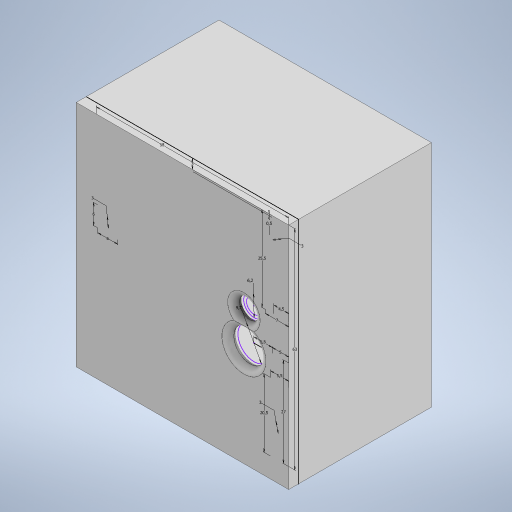
# Autodesk Inventor part: slave2
Saved by Autodesk Inventor 2023 (Build 270158000, 158)
## iProperties
Created: 2023-12-13
Part Number: slave2
Material: Generic
Document SubType Name: Modeling
Designer: magnu
Density: 1 g/cm^3
Appearance: Default
Author: magnu
Autodesk Inventor part; units mm, degrees
ref_plane "YZ Plane" through (0, 0, 0) normal (1, 0, 0) x (0, 1, 0)
ref_plane "XZ Plane" through (0, 0, 0) normal (0, 1, 0) x (-1, 0, 0)
ref_plane "XY Plane" through (0, 0, 0) normal (0, 0, 1) x (1, 0, 0)
sketch "Sketch1" plane through (0, 0, 0) normal (0, 0, 1) x (1, 0, 0)
  line L0 (0, 0) -> (58, 0)
  line L1 (58, 0) -> (58, 63)
  line L2 (58, 63) -> (0, 63)
  line L3 (0, 63) -> (0, 0)
  line L4 (0.5, 62.5) -> (57.5, 62.5)
  line L5 (57.5, 62.5) -> (57.5, 0.5)
  line L6 (57.5, 0.5) -> (0.5, 0.5)
  line L7 (0.5, 0.5) -> (0.5, 62.5)
  circle A0 centre (54.5, 8.5) radius 1.5
  circle A1 centre (54.5, 57.5) radius 1.5
  circle A2 centre (3.5, 36.5) radius 1.5
  line L8 (-3, 66) -> (61, 66)
  line L9 (61, 66) -> (61, -3)
  line L10 (61, -3) -> (-3, -3)
  line L11 (-3, -3) -> (-3, 66)
  line L12 (58, 63) -> (51, 63)
  line L13 (51, 63) -> (51, 37.5)
  line L14 (51, 37.5) -> (58, 37.5)
  line L15 (58, 37.5) -> (58, 63)
  line L16 (58, 0) -> (52.5, 0)
  line L17 (52.5, 0) -> (52.5, 20.5)
  line L18 (52.5, 20.5) -> (58, 20.5)
  line L19 (58, 20.5) -> (58, 0)
  line L20 (58, 20.5) -> (53.5, 20.5)
  line L21 (53.5, 20.5) -> (53.5, 37.5)
  line L22 (53.5, 37.5) -> (58, 37.5)
  line L23 (58, 37.5) -> (58, 20.5)
  line L24 (58, 0) -> (58, 27)
  line L25 (58, 27) -> (53, 27)
  line L26 (53, 27) -> (47.5, 27)
  circle A3 centre (47.5, 36.75) radius 2.25
  line L27 (51, 37.5) -> (51, 32.1962)
  line L28 (51, 21.8038) -> (52.5, 20.5)
  circle A4 centre (47.5, 27) radius 4.85
  circle A5 centre (47.5, 36.75) radius 3.1
  circle A6 centre (47.5, 27) radius 6
  line L29 (51, 34.1296) -> (51, 31.8734)
  line L30 (51, 21.8038) -> (50.7926, 21.9841)
  line L31 (6.5, 39.5) -> (0.5, 39.5)
  line L32 (0.5, 39.5) -> (0.5, 33.5)
  line L33 (0.5, 33.5) -> (6.5, 33.5)
  line L34 (6.5, 33.5) -> (6.5, 39.5)
  line L35 (6.5, 39.5) -> (0.5, 33.5) construction
  line L36 (0.5, 39.5) -> (6.5, 33.5) construction
  line L37 (6.5, 39.5) -> (0, 39.5)
  line L38 (0, 39.5) -> (0, 33.5)
  line L39 (0, 33.5) -> (6.5, 33.5)
  line L40 (6.5, 33.5) -> (6.5, 39.5)
  point P0 (52.5, 0.5)
  point P1 (51, 62.5)
  point P2 (50.5, 37.531)
  point P3 (50.5, 35.969)
  point P4 (57.5, 20.5)
  point P5 (57.5, 37.5)
  dimension "d0" = 58
  dimension "d1" = 63
  dimension "d2" = 0.5
  dimension "d3" = 3
  dimension "d4" = 3
  dimension "d5" = 3
  dimension "d6" = 3
  dimension "d11" = 7
  dimension "d12" = 25.5
  dimension "d13" = 5.5
  dimension "d14" = 20.5
  dimension "d15" = 4.5
  dimension "d16" = 27
  dimension "d17" = 5
  dimension "d18" = 5.5
  dimension "d25" = 9.7
  dimension "d26" = 6.2
  dimension "d31" = 6
  dimension "d32" = 6
  constraints: 82 end point, 16 parallel, 9 perpendicular, 8 point on line, 7 centre point, 6 horizontal, 2 coincident, 2 midpoint, 2 point on circle, 1 vertical, 6 other
  measures "d0" distance of L2.end L1.end
  measures "d1" distance of L1.end L0.end
  measures "d2" distance between parallel lines of L2 L4
  measures "d3" diameter of A0
  measures "d4" diameter of A1
  measures "d5" diameter of A2
  measures "d6" distance between parallel lines of L2 L8
  measures "d11" distance of L14.end L13.end
  measures "d12" distance of L13.end L12.end
  measures "d13" distance of L17.end L18.end
  measures "d14" distance of L16.end L17.end
  measures "d15" distance of L21.end L22.end
  measures "d16" distance of L0.end L24.end
  measures "d17" distance of L24.end L25.end
  measures "d18" distance of L25.end L26.end
  measures "d25" diameter of A4
  measures "d26" diameter of A5
  measures "d31" distance of L33.end L32.end
  measures "d32" distance of L32.end L31.end
extrude "Extrusion1" add sketch "Sketch1" against normal blind 40 contours L8 L9 L10 L11
extrude "Extrusion2" add sketch "Sketch1" along normal blind 3 contours L3 L39 L7 L6 L17 L0 | L17 L6 L5 L18 L1 L0 | L3 L37 L7 L39 | L17 L18 L5 L6 | L6 L7 L33 L34 L31 L4 L13 L27 L29 A6 L30 L28 L17 | L3 L2 L13 L4 L7 L37 | L7 L31 L34 L33 | L18 L5 L25 L1 | L28 L30 A6 L21 L18 | L25 L5 L14 L1 | L18 L21 L25 L5 | L2 L1 L14 L5 L4 L13 | L25 L21 L14 L5 | A6 L29 L27 L14 L21 | A6 | L4 L5 L14 L13 | A0 | A1 | A2 | L8 L9 L10 L11 | A3 | A4 | A5
extrude "Extrusion3" add sketch "Sketch1" against normal blind 5.5 contours L17 L6 L5 L18 L1 L0 | L17 L18 L5 L6 | L18 L5 L25 L1 | L28 L30 A6 L21 L18 | L25 L5 L14 L1 | L18 L21 L25 L5 | L2 L1 L14 L5 L4 L13 | L25 L21 L14 L5 | A6 L29 L27 L14 L21 | L4 L5 L14 L13
extrude "Extrusion4" add sketch "Sketch1" against normal blind 2.5 contours A0 | A1
extrude "Extrusion5" cut sketch "Sketch1" along normal through all both and the other way through all contours A3 | A4 | A5
fillet "Fillet1" radius 1.2 2 edges at (44.4, 36.75, 0) (42.65, 27, 0)
fillet "Fillet2" radius 1.79 2 edges at (44.4, 36.75, 3) (42.65, 27, 3)
body "Solid1"
